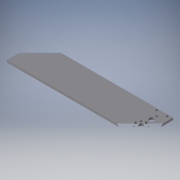
# Autodesk Inventor part: Winch Upright
Saved by Autodesk Inventor 2016 (Build 200138000, 138)
## iProperties
Created: 2015-12-16
Part Number: Winch Upright
Material: Generic
Document SubType Name: Modeling
Designer: Julia
Density: 1 g/cm^3
Appearance: Default
Author: Julia
Autodesk Inventor part; units mm, degrees
ref_plane "YZ Plane" through (0, 0, 0) normal (1, 0, 0) x (0, 1, 0)
ref_plane "XZ Plane" through (0, 0, 0) normal (0, 1, 0) x (-1, 0, 0)
ref_plane "XY Plane" through (0, 0, 0) normal (0, 0, 1) x (1, 0, 0)
sketch "Sketch1" plane through (0, 0, 0) normal (0, 1, 0) x (-1, 0, 0)
  line L0 (0, 0) -> (0, -50.8)
  line L1 (0, -50.8) -> (203.2, -50.8)
  line L2 (203.2, -50.8) -> (203.2, 0)
  line L3 (203.2, 0) -> (0, 0)
  dimension "d0" = 50.8
  dimension "d1" = 203.2
  constraints: 8 end point, 2 perpendicular, 1 horizontal, 1 vertical
  measures "d0" distance of L0.start L0.end
  measures "d1" distance of L0.end L1.end
extrude "Extrusion1" add sketch "Sketch1" along normal blind 3.302
sketch "Sketch2" plane through (0, 0, 0) normal (0, -1, 0) x (1, 0, 0)
  line L0 (-0.5, 0) -> (-0.5, -416) projected
  line L1 (-27.5, -416) -> (-0.5, -416) projected
  arc A0 (-30, -413.5) -> (-27.5, -416) centre (-27.5, -413.5) ccw projected
  line L2 (-30, -413.5) -> (-30, -2.5) projected
  arc A1 (-27.5, 0) -> (-30, -2.5) centre (-27.5, -2.5) ccw projected
  line L3 (-27.5, 0) -> (-0.5, 0) projected
  circle A2 centre (-14, -288) radius 4 projected
  circle A3 centre (-14, -320) radius 4 projected
  circle A4 centre (-14, -352) radius 4 projected
  circle A5 centre (-14, -384) radius 4 projected
  circle A6 centre (-14, -16) radius 4 projected
  circle A7 centre (-22, -16) radius 1.85 projected
  circle A8 centre (-6, -16) radius 1.85 projected
  circle A9 centre (-14, -24) radius 1.85 projected
  circle A10 centre (-14, -8) radius 1.85 projected
  circle A11 centre (-19.6569, -21.6569) radius 1.85 projected
  circle A12 centre (-19.6569, -10.3431) radius 1.85 projected
  circle A13 centre (-8.3431, -10.3431) radius 1.85 projected
  circle A14 centre (-8.3431, -21.6569) radius 1.85 projected
  circle A15 centre (-14, -80) radius 4 projected
  circle A16 centre (-22, -80) radius 1.85 projected
  circle A17 centre (-6, -80) radius 1.85 projected
  circle A18 centre (-14, -88) radius 1.85 projected
  circle A19 centre (-14, -72) radius 1.85 projected
  circle A20 centre (-19.6569, -85.6569) radius 1.85 projected
  circle A21 centre (-19.6569, -74.3431) radius 1.85 projected
  circle A22 centre (-8.3431, -74.3431) radius 1.85 projected
  circle A23 centre (-8.3431, -85.6569) radius 1.85 projected
  circle A24 centre (-14, -144) radius 4 projected
  circle A25 centre (-22, -144) radius 1.85 projected
  circle A26 centre (-6, -144) radius 1.85 projected
  circle A27 centre (-14, -152) radius 1.85 projected
  circle A28 centre (-14, -136) radius 1.85 projected
  circle A29 centre (-19.6569, -149.6569) radius 1.85 projected
  circle A30 centre (-19.6569, -138.3431) radius 1.85 projected
  circle A31 centre (-8.3431, -138.3431) radius 1.85 projected
  circle A32 centre (-8.3431, -149.6569) radius 1.85 projected
  circle A33 centre (-14, -208) radius 4 projected
  circle A34 centre (-22, -208) radius 1.85 projected
  circle A35 centre (-6, -208) radius 1.85 projected
  circle A36 centre (-14, -216) radius 1.85 projected
  circle A37 centre (-14, -200) radius 1.85 projected
  circle A38 centre (-19.6569, -213.6569) radius 1.85 projected
  circle A39 centre (-19.6569, -202.3431) radius 1.85 projected
  circle A40 centre (-8.3431, -202.3431) radius 1.85 projected
  circle A41 centre (-8.3431, -213.6569) radius 1.85 projected
  circle A42 centre (-14, -272) radius 4 projected
  circle A43 centre (-22, -272) radius 1.85 projected
  circle A44 centre (-6, -272) radius 1.85 projected
  circle A45 centre (-14, -280) radius 1.85 projected
  circle A46 centre (-14, -264) radius 1.85 projected
  circle A47 centre (-19.6569, -277.6569) radius 1.85 projected
  circle A48 centre (-19.6569, -266.3431) radius 1.85 projected
  circle A49 centre (-8.3431, -266.3431) radius 1.85 projected
  circle A50 centre (-8.3431, -277.6569) radius 1.85 projected
  circle A51 centre (-14, -336) radius 4 projected
  circle A52 centre (-22, -336) radius 1.85 projected
  circle A53 centre (-6, -336) radius 1.85 projected
  circle A54 centre (-14, -344) radius 1.85 projected
  circle A55 centre (-14, -328) radius 1.85 projected
  circle A56 centre (-19.6569, -341.6569) radius 1.85 projected
  circle A57 centre (-19.6569, -330.3431) radius 1.85 projected
  circle A58 centre (-8.3431, -330.3431) radius 1.85 projected
  circle A59 centre (-8.3431, -341.6569) radius 1.85 projected
  circle A60 centre (-14, -400) radius 4 projected
  circle A61 centre (-22, -400) radius 1.85 projected
  circle A62 centre (-6, -400) radius 1.85 projected
  circle A63 centre (-14, -408) radius 1.85 projected
  circle A64 centre (-14, -392) radius 1.85 projected
  circle A65 centre (-19.6569, -405.6569) radius 1.85 projected
  circle A66 centre (-19.6569, -394.3431) radius 1.85 projected
  circle A67 centre (-8.3431, -394.3431) radius 1.85 projected
  circle A68 centre (-8.3431, -405.6569) radius 1.85 projected
  circle A69 centre (-14, -48) radius 4 projected
  circle A70 centre (-22, -48) radius 1.85 projected
  circle A71 centre (-14, -56) radius 1.85 projected
  circle A72 centre (-6, -48) radius 1.85 projected
  circle A73 centre (-14, -40) radius 1.85 projected
  circle A74 centre (-14, -112) radius 4 projected
  circle A75 centre (-22, -112) radius 1.85 projected
  circle A76 centre (-14, -120) radius 1.85 projected
  circle A77 centre (-6, -112) radius 1.85 projected
  circle A78 centre (-14, -104) radius 1.85 projected
  circle A79 centre (-14, -176) radius 4 projected
  circle A80 centre (-22, -176) radius 1.85 projected
  circle A81 centre (-14, -184) radius 1.85 projected
  circle A82 centre (-6, -176) radius 1.85 projected
  circle A83 centre (-14, -168) radius 1.85 projected
  circle A84 centre (-14, -240) radius 4 projected
  circle A85 centre (-22, -240) radius 1.85 projected
  circle A86 centre (-14, -248) radius 1.85 projected
  circle A87 centre (-6, -240) radius 1.85 projected
  circle A88 centre (-14, -232) radius 1.85 projected
  circle A89 centre (-14, -304) radius 4 projected
  circle A90 centre (-22, -304) radius 1.85 projected
  circle A91 centre (-14, -312) radius 1.85 projected
  circle A92 centre (-6, -304) radius 1.85 projected
  circle A93 centre (-14, -296) radius 1.85 projected
  circle A94 centre (-14, -368) radius 4 projected
  circle A95 centre (-22, -368) radius 1.85 projected
  circle A96 centre (-14, -376) radius 1.85 projected
  circle A97 centre (-6, -368) radius 1.85 projected
  circle A98 centre (-14, -360) radius 1.85 projected
  circle A99 centre (-14, -32) radius 4 projected
  circle A100 centre (-14, -64) radius 4 projected
  circle A101 centre (-14, -96) radius 4 projected
  circle A102 centre (-14, -128) radius 4 projected
  circle A103 centre (-14, -160) radius 4 projected
  circle A104 centre (-14, -192) radius 4 projected
  circle A105 centre (-14, -224) radius 4 projected
  circle A106 centre (-14, -256) radius 4 projected
  point P0 (0, 0)
extrude "Extrusion2" cut sketch "Sketch2" against normal blind 20.5105 contours A6 | A7 | A8 | A9 | A10 | A11 | A12 | A13 | A14 | A70 | A72 | A73 | A99
body "Solid1"
